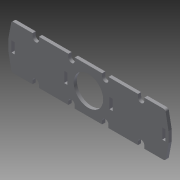
# Autodesk Inventor part: Camera Platform
Saved by Autodesk Inventor 2013 (Build 170138000, 138)
## iProperties
Created: 2013-05-28
Part Number: Camera Platform
Material: Generic
Document SubType Name: Modeling
Designer: Eric
Density: 1 g/cm^3
Author: Eric
Autodesk Inventor part; units mm, degrees
ref_plane "YZ Plane" through (0, 0, 0) normal (1, 0, 0) x (0, 1, 0)
ref_plane "XZ Plane" through (0, 0, 0) normal (0, 1, 0) x (-1, 0, 0)
ref_plane "XY Plane" through (0, 0, 0) normal (0, 0, 1) x (1, 0, 0)
sketch "Sketch1" plane through (0, 0, 0) normal (0, 1, 0) x (-1, 0, 0)
  line L0 (76, -4.8141) -> (76, 4.8141)
  line L1 (-76, 4.8141) -> (-76, -4.8141)
  circle A0 centre (0, 0) radius 14
  line L2 (-23, 5) -> (-20, 5)
  line L3 (-20, 5) -> (-20, -5)
  line L4 (-20, -5) -> (-23, -5)
  line L5 (-23, -5) -> (-23, 5)
  line L6 (20, 5) -> (23, 5)
  line L7 (23, 5) -> (23, -5)
  line L8 (23, -5) -> (20, -5)
  line L9 (20, -5) -> (20, 5)
  line L10 (-73, 5) -> (-70, 5)
  line L11 (-70, 5) -> (-70, -5)
  line L12 (-70, -5) -> (-73, -5)
  line L13 (-73, -5) -> (-73, 5)
  line L14 (70, 5) -> (73, 5)
  line L15 (73, 5) -> (73, -5)
  line L16 (73, -5) -> (70, -5)
  line L17 (70, -5) -> (70, 5)
  arc A1 (-13, -18) -> (-19, -18) centre (-16, -18) ccw
  arc A2 (-19, 18) -> (-13, 18) centre (-16, 18) ccw
  arc A3 (19, -18) -> (13, -18) centre (16, -18) ccw
  arc A4 (13, 18) -> (19, 18) centre (16, 18) ccw
  line L18 (-19, 18) -> (-19, 21)
  line L19 (-13, 18) -> (-13, 21)
  line L20 (13, 18) -> (13, 21)
  line L21 (19, 18) -> (19, 21)
  line L22 (13, -18) -> (13, -21)
  line L23 (19, -18) -> (19, -21)
  line L24 (-13, -18) -> (-13, -21)
  line L25 (-19, -18) -> (-19, -21)
  line L26 (-13, -21) -> (13, -21)
  line L27 (13, 21) -> (-13, 21)
  arc A5 (-53, 18) -> (-47, 18) centre (-50, 18) ccw
  arc A6 (-47, -18) -> (-53, -18) centre (-50, -18) ccw
  arc A7 (47, 18) -> (53, 18) centre (50, 18) ccw
  arc A8 (53, -18) -> (47, -18) centre (50, -18) ccw
  line L28 (-53, 18) -> (-53, 21)
  line L29 (-47, 18) -> (-47, 21)
  line L30 (-53, -18) -> (-53, -21)
  line L31 (-47, -18) -> (-47, -21)
  line L32 (53, -18) -> (53, -21)
  line L33 (47, -18) -> (47, -21)
  line L34 (53, 18) -> (53, 21)
  line L35 (47, 18) -> (47, 21)
  line L36 (71.3401, 21) -> (53, 21)
  line L37 (47, 21) -> (19, 21)
  line L38 (19, -21) -> (47, -21)
  line L39 (53, -21) -> (71.3401, -21)
  line L40 (-71.3401, -21) -> (-53, -21)
  line L41 (-47, -21) -> (-19, -21)
  line L42 (-19, 21) -> (-47, 21)
  line L43 (-53, 21) -> (-71.3401, 21)
  line L44 (-75.9657, 5.1827) -> (-73.3059, 19.3686)
  line L45 (-73.3059, -19.3686) -> (-75.9657, -5.1827)
  line L46 (73.3059, 19.3686) -> (75.9657, 5.1827)
  line L47 (73.3059, -19.3686) -> (75.9657, -5.1827)
  arc A9 (-71.3401, 21) -> (-73.3059, 19.3686) centre (-71.3401, 19) ccw
  arc A10 (-75.9657, 5.1827) -> (-76, 4.8141) centre (-74, 4.8141) ccw
  arc A11 (-76, -4.8141) -> (-75.9657, -5.1827) centre (-74, -4.8141) ccw
  arc A12 (-73.3059, -19.3686) -> (-71.3401, -21) centre (-71.3401, -19) ccw
  arc A13 (71.3401, -21) -> (73.3059, -19.3686) centre (71.3401, -19) ccw
  arc A14 (75.9657, -5.1827) -> (76, -4.8141) centre (74, -4.8141) ccw
  arc A15 (73.3059, 19.3686) -> (71.3401, 21) centre (71.3401, 19) ccw
  arc A16 (76, 4.8141) -> (75.9657, 5.1827) centre (74, 4.8141) ccw
  point P0 (-73, -21)
  point P1 (73, 21)
  point P2 (73, -21)
  point P3 (-73, 21)
  point P4 (-20, 0)
  point P5 (20, 0)
  point P6 (-76, 5)
  point P7 (-76, -5)
  point P8 (76, 5)
  point P9 (76, -5)
  dimension "d2" = 42
  dimension "d3" = 28
  dimension "d4" = 76
  dimension "d6" = 3
  dimension "d7" = 10
  dimension "d8" = 20
  dimension "d9" = 3
  dimension "d10" = 10
  dimension "d11" = 20
  dimension "d12" = 3
  dimension "d13" = 10
  dimension "d14" = 3
  dimension "d15" = 3
  dimension "d16" = 10
  dimension "d17" = 3
  dimension "d18" = 5
  dimension "d19" = 5
  dimension "d20" = 6
  dimension "d21" = 16
  dimension "d24" = 6
  dimension "d25" = 16
  dimension "d26" = 6
  dimension "d27" = 16
  dimension "d28" = 6
  dimension "d29" = 16
  dimension "d32" = 6
  dimension "d33" = 50
  dimension "d35" = 50
  dimension "d38" = 76
  dimension "d39" = 21
  dimension "d40" = 3
  dimension "d41" = 3
  dimension "d42" = 10
  dimension "d43" = 10
  dimension "d44" = 21
  dimension "d45" = 2
  dimension "d46" = 50
  dimension "d47" = 50
  dimension "d48" = 3
  dimension "d49" = 3
  dimension "d50" = 3
  dimension "d51" = 3
  dimension "d52" = 3
  dimension "d53" = 3
  dimension "d54" = 3
  dimension "d55" = 3
  dimension "d56" = 100.62
  constraints: 96 end point, 54 perpendicular, 40 parallel, 38 tangent, 32 point on circle, 17 centre point, 16 point on line, 9 horizontal, 7 equal radius, 5 collinear, 2 coincident, 2 horizontal alignment, 2 midpoint
  measures "d2" distance of point (-73, 21) point (-73, -21)
  measures "d3" diameter of A0
  measures "d4" distance from line of L1 A0.centre
  measures "d6" distance of L3.end L4.end
  measures "d7" distance of L2.end L3.end
  measures "d8" distance from line of point (0, 0) L3
  measures "d9" distance of L7.end L8.end
  measures "d10" distance of L6.end L7.end
  measures "d11" distance from line of point (0, 0) L9
  measures "d12" distance of L10.start L10.end
  measures "d13" distance of L10.end L11.end
  measures "d14" distance between parallel lines of L1 L13
  measures "d15" distance of L14.start L14.end
  measures "d16" distance of L16.end L14.start
  measures "d17" distance between parallel lines of L0 L15
  measures "d18" distance from line of point (0, 0) L14
  measures "d19" distance from line of point (0, 0) L10
  measures "d20" diameter of A1
  measures "d21" horizontal distance of point (0, 0) A1.centre
  measures "d24" diameter of A2
  measures "d25" horizontal distance of point (0, 0) A2.centre
  measures "d26" diameter of A3
  measures "d27" horizontal distance of point (0, 0) A3.centre
  measures "d28" diameter of A4
  measures "d29" horizontal distance of point (0, 0) A4.centre
  measures "d32" diameter of A5
  measures "d33" horizontal distance of point (0, 0) A5.centre
  measures "d35" horizontal distance of point (0, 0) A7.centre
  measures "d38" distance from line of point (0, 0) L0
  measures "d39" distance from line of point (0, 0) L43
  measures "d40" distance from line of point (-73, 21) L1
  measures "d41" horizontal distance of point (76, 5) point (73, 21)
  measures "d42" distance of point (76, -5) point (76, 5)
  measures "d43" distance of point (-76, 5) point (-76, -5)
  measures "d44" distance from line of point (0, 0) L40
  measures "d45" radius of A9
  measures "d46" horizontal distance of point (0, 0) A6.centre
  measures "d47" horizontal distance of A8.centre point (0, 0)
  measures "d48" distance from line of L42 A5.centre
  measures "d49" distance from line of L37 A7.centre
  measures "d50" distance from line of L38 A8.centre
  measures "d51" distance from line of L41 A6.centre
  measures "d52" distance from line of L41 A1.centre
  measures "d53" distance from line of L38 A3.centre
  measures "d54" distance from line of A2.centre L42
  measures "d55" distance from line of L37 A4.centre
  measures "d56" angle of L43 L44
extrude "Extrusion1" add sketch "Sketch1" along normal blind 3
body "Solid1"
